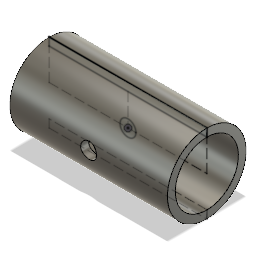
Table_17p1_Problem_18 (Autodesk Fusion 360 design; units mm, degrees)
Autodesk Fusion 360 part; units mm, degrees
sketch "Sketch1" plane through (0, 0, 0) normal (0, 0, 1) x (1, 0, 0)
  line L0 (-100, 50) -> (100, 50)
  line L1 (100, 50) -> (100, 40)
  line L2 (100, 40) -> (-100, 40)
  line L3 (-100, 40) -> (-100, 50)
  line L4 (0, 40) -> (0, 0) construction
  line L5 (-100, 0) -> (100, 0) construction
  line L6 (100, 0) -> (100, 40) construction
  line L7 (-100, 0) -> (-100, 40) construction
  line L8 (-100, -50) -> (100, -50) construction
  line L9 (100, -40) -> (-100, -40) construction
  line L10 (100, -50) -> (100, -40) construction
  line L11 (-100, -40) -> (-100, -50) construction
  circle A0 centre (0, 0) radius 10
  dimension "Inner_Diameter" = 80
  dimension "Outer_Diameter" = 100
  dimension "Bar_Length" = 200
  dimension "Hole_Radius" = 10
  constraint coincident L4.end A0.centre
  constraint horizontal L0
  constraint vertical L1
  constraint horizontal L2
  constraint vertical L3
  constraint midpoint L2 L4.start
  constraint vertical L4
  constraint horizontal L5
  constraint vertical L7
  constraint vertical L6
  constraint coincident L4.end L5
  constraint symmetric L0.start L5 L8.start
  constraint symmetric L0.end L5 L8.end
  constraint symmetric L1.end L5 L9.start
  constraint symmetric L2.end L5 L9.end
  measures "Inner_Diameter" distance of L2 L9
  measures "Outer_Diameter" distance of L0 L8
  measures "Bar_Length" distance of L0.start L0.end
  measures "Hole_Radius" radius of A0
revolve "Revolve1" add sketch "Sketch1" angle 360 about axis through (-100, 0, 0) along (1, 0, 0) contours L0 L1 L2 L3
extrude "Extrude1" cut sketch "Sketch1" along normal through all contours A0
